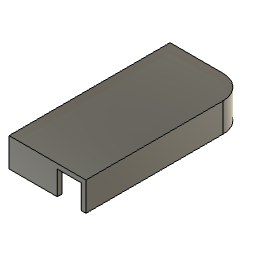
model (Autodesk Fusion 360 design; units mm, degrees)
Autodesk Fusion 360 part; units mm, degrees
sketch "Sketch1" plane through (0, 0, 0) normal (0, 0, 1) x (1, 0, 0)
  line L0 (0, 0) -> (155, 0)
  line L1 (155, 0) -> (155, 311)
  line L2 (155, 311) -> (0, 311)
  line L3 (0, 311) -> (0, 0)
  dimension "d1" = 155
  dimension "d2" = 311
  constraint horizontal L0
  constraint vertical L1
  constraint horizontal L2
  constraint vertical L3
  constraint coincident L0.start L3.end
  measures "d1" distance of L0.start L0.end
  measures "d2" distance of L0.start L2.end
extrude "Extrude1" add sketch "Sketch1" along normal blind 60
fillet "Fillet1" radius 50 1 edges at (155, 311, 30)
move_face "OffsetFaces1" offset 10 1 faces at (51.6667, 0, 20)
move_face "OffsetFaces2" offset 5 1 faces at (0, 204, 40)
shell "Shell1" thickness 10 removed faces 1 at (48.3333, 187.3333, 0)
sketch "Sketch2" plane through (0, -10, 0) normal (0, -1, 0) x (1, 0, 0)
  line L0 (-5, 0) -> (155, 0)
  line L1 (155, 0) -> (155, 60)
  line L2 (155, 60) -> (-5, 60)
  line L3 (-5, 60) -> (-5, 0)
  line L4 (105.387, 60) -> (160.387, 60)
  line L5 (160.387, 60) -> (160.387, 0)
  line L6 (160.387, 0) -> (105.387, 0)
  line L7 (105.387, 0) -> (105.387, 60)
  dimension "d10" = 55
  dimension "d11" = 60
  constraint horizontal L4
  constraint vertical L5
  constraint horizontal L6
  constraint vertical L7
  constraint coincident L2 L4.start
  measures "d10" distance of L4.start L4.end
  measures "d11" distance of L4.start L6.end
extrude "Extrude2" cut sketch "Sketch2" against normal blind 10 contours L0 L1 L2 L4 L6 L7
sketch "Sketch3" plane through (0, 0, 0) normal (0, 0, 1) x (1, 0, 0)
  line L0 (145, 0) -> (155, 0)
  line L1 (155, 0) -> (155, -10)
  line L2 (155, -10) -> (145, -10)
  line L3 (145, -10) -> (145, 0)
  point P0 (145, 0)
  dimension "d14" = 10
  constraint horizontal L0
  constraint vertical L1
  constraint horizontal L2
  constraint vertical L3
  constraint coincident P0 L0.start
  measures "d14" distance of P0 L2.end
extrude "Extrude3" add sketch "Sketch3" along normal blind 60
sketch "Sketch4" plane through (0, 0, 0) normal (0, 0, 1) x (1, 0, 0)
  line L0 (145, 0, 60) -> (105, 0, 60)
  line L1 (105, 0, 60) -> (105, 0, 50)
  line L2 (105, 0, 50) -> (145, 0, 50)
  line L3 (145, 0, 50) -> (145, 0, 60)
  point P0 (145, 0)
  dimension "d17" = 40
  dimension "d18" = 10
extrude "Extrude4" add sketch "Sketch4" against normal blind 10 contours L0 L1 L2 L3 in plane through (0, 0, 0) normal (0, 1, 0)
sketch "Sketch5" plane through (105.387, 0, 0) normal (1, 0, 0) x (0, 1, 0)
  line L0 (0, 50) -> (-10, 50)
  line L1 (-10, 50) -> (-10, 0)
  line L2 (-10, 0) -> (0, 0)
  line L3 (0, 0) -> (0, 50)
  line L4 (0, 0) -> (-10, 0)
  line L5 (-10, 0, 0) -> (-10, 0, -10)
  line L6 (-10, 0, -10) -> (0, 0, -10)
  line L7 (0, 0, -10) -> (0, 0, 0)
  dimension "d21" = 10
  dimension "d22" = 10
  constraint horizontal L4
  constraint coincident L2.end L3.start
  measures "d21" distance of L2.end L1.end
  measures "d22" distance of L2.end L3.start
extrude "Extrude5" cut sketch "Sketch5" against normal blind 50 contours L2 L4 L5 L6 L7 in plane through (105.387, 0, 0) normal (0, 0, 1)
sketch "Sketch6" plane through (0, 0, 50) normal (0, 0, -1) x (1, 0, 0)
  arc A0 (105, -301) -> (145, -261) centre (105, -261) ccw
  line L0 (145, -261) -> (145, 10)
  line L1 (145, 10) -> (105.387, 10)
  line L2 (105.387, 10) -> (105.387, 0)
  line L3 (105.387, 0) -> (5, 0)
  line L4 (5, 0) -> (5, -301)
  line L5 (5, -301) -> (105, -301)
  line L6 (105.387, 10, 50) -> (95.387, 10, 50)
  line L7 (95.387, 10, 50) -> (95.387, 0, 50)
  line L8 (95.387, 0, 50) -> (105.387, 0, 50)
  line L9 (105.387, 0, 50) -> (105.387, 10, 50)
  point P0 (105.387, 10)
  dimension "d25" = 10
  dimension "d26" = 10
  constraint coincident P0 L1.end
  measures "d26" distance of P0 L2.end
extrude "Extrude6" cut sketch "Sketch6" against normal blind 50 contours L6 L7 L8 L9 in plane through (0, 0, 0) normal (0, 0, -1)
move_face "OffsetFaces3" offset 9 1 faces at (28.4623, -10, 36.6667)
sketch "Sketch7" plane through (0, 0, 0) normal (0, 0, -1) x (1, 0, 0)
  line L0 (95.387, 0) -> (95.387, 19)
  line L1 (95.387, 19) -> (-5, 19)
  line L2 (-5, 19) -> (-5, -311)
  line L3 (-5, -311) -> (105, -311)
  arc A0 (105, -311) -> (155, -261) centre (105, -261) ccw
  line L4 (155, -261) -> (155, 19)
  line L5 (155, 19) -> (145, 19)
  line L6 (145, 19) -> (145, -261)
  arc A1 (105, -301) -> (145, -261) centre (105, -261) ccw
  line L7 (105, -301) -> (5, -301)
  line L8 (5, -301) -> (5, 0)
  line L9 (5, 0) -> (95.387, 0)
  line L10 (95.387, 0) -> (5.387, 0)
  line L11 (5.387, 0) -> (5.387, 9)
  line L12 (5.387, 9) -> (95.387, 9)
  line L13 (95.387, 9) -> (95.387, 0)
  dimension "d30" = 90
  dimension "d31" = 9
  constraint horizontal L10
  constraint vertical L11
  constraint horizontal L12
  constraint vertical L13
  constraint coincident L0.start L9.end
  measures "d30" distance of L0.start L10.end
  measures "d31" distance of L0.start L12.end
extrude "Extrude7" cut sketch "Sketch7" against normal blind 50 contours L0 L9 L10 L11 L12 L13
sketch "Sketch8" plane through (0, 0, 0) normal (0, 0, 1) x (1, 0, 0)
  line L0 (5.4, -9) -> (5, -9)
  line L1 (5, -9) -> (5, 0)
  line L2 (5, 0) -> (5.4, 0)
  line L3 (5.4, 0) -> (5.4, -9)
  constraint horizontal L0
  constraint vertical L1
  constraint horizontal L2
  constraint vertical L3
extrude "Extrude8" cut sketch "Sketch8" along normal blind 50
sketch "Sketch9" plane through (0, 0, 50) normal (0, 0, -1) x (1, 0, 0)
  line L0 (95.387, 9) -> (5, 9)
  line L1 (5, 9) -> (5, -301)
  line L2 (5, -301) -> (105, -301)
  arc A0 (105, -301) -> (145, -261) centre (105, -261) ccw
  line L3 (145, -261) -> (145, 19)
  line L4 (145, 19) -> (95.387, 19)
  line L5 (95.387, 19) -> (95.387, 9)
move_face "OffsetFaces4" offset 5 1 faces at (28.4623, -19, 36.6667)
sketch "Sketch10" plane through (0, 0, 0) normal (0, 0, -1) x (1, 0, 0)
  line L0 (5, -301) -> (5, 9)
  line L1 (5, 9) -> (95.387, 9)
  line L2 (95.387, 9) -> (95.387, 24)
  line L3 (95.387, 24) -> (-5, 24)
  line L4 (-5, 24) -> (-5, -311)
  line L5 (-5, -311) -> (105, -311)
  arc A0 (105, -311) -> (155, -261) centre (105, -261) ccw
  line L6 (155, -261) -> (155, 24)
  line L7 (155, 24) -> (145, 24)
  line L8 (145, 24) -> (145, -261)
  arc A1 (105, -301) -> (145, -261) centre (105, -261) ccw
  line L9 (105, -301) -> (5, -301)
  line L10 (5, 9) -> (95.387, 9)
  line L11 (95.387, 9) -> (95.387, 14)
  line L12 (95.387, 14) -> (5, 14)
  line L13 (5, 14) -> (5, 9)
  dimension "d37" = 5
  constraint horizontal L10
  constraint vertical L11
  constraint horizontal L12
  constraint vertical L13
  constraint coincident L0.end L1.start
  measures "d37" distance of L0.end L12.end
extrude "Extrude9" cut sketch "Sketch10" against normal blind 50 contours L1 L2 L10 L11 L12 L13
